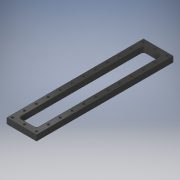
# Autodesk Inventor part: PVCmiddle
Saved by Autodesk Inventor 2019.4 (Build 234330000, 330)
## iProperties
Created: 2020-04-27
Part Number: PVCmiddle
Material: Generic
Document SubType Name: Modeling
Designer: Ed
Density: 1 g/cm^3
Appearance: Default
Author: Ed
Autodesk Inventor part; units mm, degrees
ref_plane "YZ Plane" through (0, 0, 0) normal (1, 0, 0) x (0, 1, 0)
ref_plane "XZ Plane" through (0, 0, 0) normal (0, 1, 0) x (-1, 0, 0)
ref_plane "XY Plane" through (0, 0, 0) normal (0, 0, 1) x (1, 0, 0)
sketch "Sketch1" plane through (0, 0, 0) normal (0, 1, 0) x (-1, 0, 0)
  line L0 (135.3948, 0) -> (136.2838, 0)
  arc A0 (162.481, 269.4826) -> (164.973, 271.8943) centre (162.56, 271.8943) ccw
  arc A1 (164.973, 271.8943) -> (164.8183, 272.7443) centre (162.56, 271.8943) ccw
  arc A2 (164.8183, 272.7443) -> (163.1941, 274.2225) centre (162.56, 271.8943) ccw
  arc A3 (163.1941, 274.2225) -> (162.7264, 274.3016) centre (162.56, 271.8943) ccw
  arc A4 (162.7264, 274.3016) -> (160.2292, 272.5188) centre (162.56, 271.8943) ccw
  arc A5 (160.2292, 272.5188) -> (160.147, 271.8943) centre (162.56, 271.8943) ccw
  arc A6 (160.147, 271.8943) -> (161.9355, 269.5635) centre (162.56, 271.8943) ccw
  arc A7 (161.9355, 269.5635) -> (162.481, 269.4826) centre (162.56, 271.8943) ccw
  arc A8 (162.3235, 242.9385) -> (164.2662, 243.6336) centre (162.56, 245.3399) ccw
  arc A9 (164.2662, 243.6336) -> (164.973, 245.3399) centre (162.56, 245.3399) ccw
  arc A10 (164.973, 245.3399) -> (162.7965, 247.7413) centre (162.56, 245.3399) ccw
  arc A11 (162.7965, 247.7413) -> (160.8538, 247.0461) centre (162.56, 245.3399) ccw
  arc A12 (160.8538, 247.0461) -> (160.147, 245.3399) centre (162.56, 245.3399) ccw
  arc A13 (160.147, 245.3399) -> (162.3235, 242.9385) centre (162.56, 245.3399) ccw
  arc A14 (162.481, 216.3737) -> (164.973, 218.7854) centre (162.56, 218.7854) ccw
  arc A15 (164.973, 218.7854) -> (164.8691, 219.4859) centre (162.56, 218.7854) ccw
  arc A16 (164.8691, 219.4859) -> (163.1463, 221.1261) centre (162.56, 218.7854) ccw
  arc A17 (163.1463, 221.1261) -> (162.5304, 221.1983) centre (162.56, 218.7854) ccw
  arc A18 (162.5304, 221.1983) -> (160.8538, 220.4917) centre (162.56, 218.7854) ccw
  arc A19 (160.8538, 220.4917) -> (160.147, 218.7854) centre (162.56, 218.7854) ccw
  arc A20 (160.147, 218.7854) -> (161.9355, 216.4547) centre (162.56, 218.7854) ccw
  arc A21 (161.9355, 216.4547) -> (162.481, 216.3737) centre (162.56, 218.7854) ccw
  arc A22 (162.3235, 189.8296) -> (164.2662, 190.5248) centre (162.56, 192.231) ccw
  arc A23 (164.2662, 190.5248) -> (164.973, 192.231) centre (162.56, 192.231) ccw
  arc A24 (164.973, 192.231) -> (163.1845, 194.5618) centre (162.56, 192.231) ccw
  arc A25 (163.1845, 194.5618) -> (162.7178, 194.6388) centre (162.56, 192.231) ccw
  arc A26 (162.7178, 194.6388) -> (161.3535, 194.3207) centre (162.56, 192.231) ccw
  arc A27 (161.3535, 194.3207) -> (160.147, 192.231) centre (162.56, 192.231) ccw
  arc A28 (160.147, 192.231) -> (162.3235, 189.8296) centre (162.56, 192.231) ccw
  arc A29 (162.481, 163.2649) -> (164.973, 165.6766) centre (162.56, 165.6766) ccw
  arc A30 (164.973, 165.6766) -> (164.6497, 166.8831) centre (162.56, 165.6766) ccw
  arc A31 (164.6497, 166.8831) -> (162.7178, 168.0844) centre (162.56, 165.6766) ccw
  arc A32 (162.7178, 168.0844) -> (161.3535, 167.7663) centre (162.56, 165.6766) ccw
  arc A33 (161.3535, 167.7663) -> (160.147, 165.6766) centre (162.56, 165.6766) ccw
  arc A34 (160.147, 165.6766) -> (161.9355, 163.3458) centre (162.56, 165.6766) ccw
  arc A35 (161.9355, 163.3458) -> (162.481, 163.2649) centre (162.56, 165.6766) ccw
  arc A36 (162.3235, 136.7208) -> (164.2662, 137.4159) centre (162.56, 139.1221) ccw
  arc A37 (164.2662, 137.4159) -> (164.973, 139.1222) centre (162.56, 139.1221) ccw
  arc A38 (164.973, 139.1222) -> (163.1845, 141.4529) centre (162.56, 139.1221) ccw
  arc A39 (163.1845, 141.4529) -> (162.7178, 141.53) centre (162.56, 139.1221) ccw
  arc A40 (162.7178, 141.53) -> (161.3535, 141.2119) centre (162.56, 139.1221) ccw
  arc A41 (161.3535, 141.2119) -> (160.147, 139.1222) centre (162.56, 139.1221) ccw
  arc A42 (160.147, 139.1222) -> (162.3235, 136.7208) centre (162.56, 139.1221) ccw
  arc A43 (162.481, 110.156) -> (164.973, 112.5677) centre (162.56, 112.5677) ccw
  arc A44 (164.973, 112.5677) -> (164.7242, 113.635) centre (162.56, 112.5677) ccw
  arc A45 (164.7242, 113.635) -> (162.7572, 114.9726) centre (162.56, 112.5677) ccw
  arc A46 (162.7572, 114.9726) -> (161.9355, 114.8985) centre (162.56, 112.5677) ccw
  arc A47 (161.9355, 114.8985) -> (160.147, 112.5677) centre (162.56, 112.5677) ccw
  arc A48 (160.147, 112.5677) -> (161.9355, 110.2369) centre (162.56, 112.5677) ccw
  arc A49 (161.9355, 110.2369) -> (162.481, 110.156) centre (162.56, 112.5677) ccw
  arc A50 (162.7178, 83.6055) -> (164.6497, 84.8068) centre (162.56, 86.0133) ccw
  arc A51 (164.6497, 84.8068) -> (164.973, 86.0133) centre (162.56, 86.0133) ccw
  arc A52 (164.973, 86.0133) -> (163.0308, 88.3799) centre (162.56, 86.0133) ccw
  arc A53 (163.0308, 88.3799) -> (162.7572, 88.4182) centre (162.56, 86.0133) ccw
  arc A54 (162.7572, 88.4182) -> (161.9355, 88.3441) centre (162.56, 86.0133) ccw
  arc A55 (161.9355, 88.3441) -> (160.147, 86.0133) centre (162.56, 86.0133) ccw
  arc A56 (160.147, 86.0133) -> (161.9355, 83.6825) centre (162.56, 86.0133) ccw
  arc A57 (161.9355, 83.6825) -> (162.7178, 83.6055) centre (162.56, 86.0133) ccw
  arc A58 (162.481, 57.0472) -> (164.973, 59.4589) centre (162.56, 59.4589) ccw
  arc A59 (164.973, 59.4589) -> (164.4253, 60.9897) centre (162.56, 59.4589) ccw
  arc A60 (164.4253, 60.9897) -> (162.6192, 61.8711) centre (162.56, 59.4589) ccw
  arc A61 (162.6192, 61.8711) -> (161.9355, 61.7896) centre (162.56, 59.4589) ccw
  arc A62 (161.9355, 61.7896) -> (160.147, 59.4589) centre (162.56, 59.4589) ccw
  arc A63 (160.147, 59.4589) -> (161.9355, 57.1281) centre (162.56, 59.4589) ccw
  arc A64 (161.9355, 57.1281) -> (162.481, 57.0472) centre (162.56, 59.4589) ccw
  arc A65 (162.7178, 30.4966) -> (164.6497, 31.6979) centre (162.56, 32.9044) ccw
  arc A66 (164.6497, 31.6979) -> (164.973, 32.9044) centre (162.56, 32.9044) ccw
  arc A67 (164.973, 32.9044) -> (163.0308, 35.2711) centre (162.56, 32.9044) ccw
  arc A68 (163.0308, 35.2711) -> (162.7572, 35.3094) centre (162.56, 32.9044) ccw
  arc A69 (162.7572, 35.3094) -> (161.9355, 35.2352) centre (162.56, 32.9044) ccw
  arc A70 (161.9355, 35.2352) -> (160.147, 32.9044) centre (162.56, 32.9044) ccw
  arc A71 (160.147, 32.9044) -> (161.9355, 30.5737) centre (162.56, 32.9044) ccw
  arc A72 (161.9355, 30.5737) -> (162.7178, 30.4966) centre (162.56, 32.9044) ccw
  arc A73 (160.147, 6.35) -> (164.973, 6.35) centre (162.56, 6.35) ccw
  arc A74 (164.973, 6.35) -> (164.4253, 7.8808) centre (162.56, 6.35) ccw
  arc A75 (164.4253, 7.8808) -> (162.6192, 8.7623) centre (162.56, 6.35) ccw
  arc A76 (162.6192, 8.7623) -> (161.9355, 8.6808) centre (162.56, 6.35) ccw
  arc A77 (161.9355, 8.6808) -> (160.147, 6.35) centre (162.56, 6.35) ccw
  arc A78 (133.477, 6.35) -> (138.2208, 5.7255) centre (135.89, 6.35) ccw
  arc A79 (138.2208, 5.7255) -> (138.2824, 6.035) centre (135.89, 6.35) ccw
  arc A80 (138.2824, 6.035) -> (138.2978, 6.1922) centre (135.89, 6.35) ccw
  arc A81 (138.2978, 6.1922) -> (138.303, 6.35) centre (135.89, 6.35) ccw
  arc A82 (138.303, 6.35) -> (135.2655, 8.6808) centre (135.89, 6.35) ccw
  arc A83 (135.2655, 8.6808) -> (133.477, 6.35) centre (135.89, 6.35) ccw
  arc A84 (109.22, 8.763) -> (107.8794, 8.3563) centre (109.22, 6.35) ccw
  arc A85 (107.8794, 8.3563) -> (106.807, 6.35) centre (109.22, 6.35) ccw
  arc A86 (106.807, 6.35) -> (111.1814, 4.9445) centre (109.22, 6.35) ccw
  arc A87 (111.1814, 4.9445) -> (111.5508, 5.7255) centre (109.22, 6.35) ccw
  arc A88 (111.5508, 5.7255) -> (111.6278, 6.1922) centre (109.22, 6.35) ccw
  arc A89 (111.6278, 6.1922) -> (111.633, 6.35) centre (109.22, 6.35) ccw
  arc A90 (111.633, 6.35) -> (109.22, 8.763) centre (109.22, 6.35) ccw
  arc A91 (109.3088, 35.3158) -> (109.22, 35.3174) centre (109.22, 32.9044) ccw
  arc A92 (109.22, 35.3174) -> (106.807, 32.9044) centre (109.22, 32.9044) ccw
  arc A93 (106.807, 32.9044) -> (108.5955, 30.5737) centre (109.22, 32.9044) ccw
  arc A94 (108.5955, 30.5737) -> (109.141, 30.4927) centre (109.22, 32.9044) ccw
  arc A95 (109.141, 30.4927) -> (111.633, 32.9044) centre (109.22, 32.9044) ccw
  arc A96 (111.633, 32.9044) -> (109.6908, 35.2711) centre (109.22, 32.9044) ccw
  arc A97 (109.6908, 35.2711) -> (109.5741, 35.2913) centre (109.22, 32.9044) ccw
  arc A98 (109.5741, 35.2913) -> (109.3088, 35.3158) centre (109.22, 32.9044) ccw
  arc A99 (109.3384, 61.869) -> (109.22, 61.8719) centre (109.22, 59.4589) ccw
  arc A100 (109.22, 61.8719) -> (107.8794, 61.4652) centre (109.22, 59.4589) ccw
  arc A101 (107.8794, 61.4652) -> (106.807, 59.4589) centre (109.22, 59.4589) ccw
  arc A102 (106.807, 59.4589) -> (108.5955, 57.1281) centre (109.22, 59.4589) ccw
  arc A103 (108.5955, 57.1281) -> (109.141, 57.0472) centre (109.22, 59.4589) ccw
  arc A104 (109.141, 57.0472) -> (111.633, 59.4589) centre (109.22, 59.4589) ccw
  arc A105 (111.633, 59.4589) -> (109.6908, 61.8255) centre (109.22, 59.4589) ccw
  arc A106 (109.6908, 61.8255) -> (109.3384, 61.869) centre (109.22, 59.4589) ccw
  arc A107 (109.3088, 88.4247) -> (109.22, 88.4263) centre (109.22, 86.0133) ccw
  arc A108 (109.22, 88.4263) -> (106.807, 86.0133) centre (109.22, 86.0133) ccw
  arc A109 (106.807, 86.0133) -> (108.5955, 83.6825) centre (109.22, 86.0133) ccw
  arc A110 (108.5955, 83.6825) -> (109.141, 83.6016) centre (109.22, 86.0133) ccw
  arc A111 (109.141, 83.6016) -> (111.633, 86.0133) centre (109.22, 86.0133) ccw
  arc A112 (111.633, 86.0133) -> (109.6908, 88.3799) centre (109.22, 86.0133) ccw
  arc A113 (109.6908, 88.3799) -> (109.5741, 88.4002) centre (109.22, 86.0133) ccw
  arc A114 (109.5741, 88.4002) -> (109.3088, 88.4247) centre (109.22, 86.0133) ccw
  arc A115 (109.3384, 114.9778) -> (109.22, 114.9807) centre (109.22, 112.5677) ccw
  arc A116 (109.22, 114.9807) -> (107.5138, 114.274) centre (109.22, 112.5677) ccw
  arc A117 (107.5138, 114.274) -> (106.807, 112.5677) centre (109.22, 112.5677) ccw
  arc A118 (106.807, 112.5677) -> (108.5955, 110.2369) centre (109.22, 112.5677) ccw
  arc A119 (108.5955, 110.2369) -> (109.141, 110.156) centre (109.22, 112.5677) ccw
  arc A120 (109.141, 110.156) -> (111.633, 112.5677) centre (109.22, 112.5677) ccw
  arc A121 (111.633, 112.5677) -> (109.6908, 114.9344) centre (109.22, 112.5677) ccw
  arc A122 (109.6908, 114.9344) -> (109.3384, 114.9778) centre (109.22, 112.5677) ccw
  arc A123 (109.3088, 141.5335) -> (109.22, 141.5352) centre (109.22, 139.1222) ccw
  arc A124 (109.22, 141.5352) -> (106.807, 139.1222) centre (109.22, 139.1222) ccw
  arc A125 (106.807, 139.1222) -> (108.5955, 136.7914) centre (109.22, 139.1222) ccw
  arc A126 (108.5955, 136.7914) -> (109.141, 136.7104) centre (109.22, 139.1222) ccw
  arc A127 (109.141, 136.7104) -> (111.633, 139.1222) centre (109.22, 139.1222) ccw
  arc A128 (111.633, 139.1222) -> (109.6908, 141.4888) centre (109.22, 139.1222) ccw
  arc A129 (109.6908, 141.4888) -> (109.5741, 141.509) centre (109.22, 139.1222) ccw
  arc A130 (109.5741, 141.509) -> (109.3088, 141.5335) centre (109.22, 139.1222) ccw
  arc A131 (109.3384, 168.0867) -> (109.22, 168.0896) centre (109.22, 165.6766) ccw
  arc A132 (109.22, 168.0896) -> (107.5138, 167.3828) centre (109.22, 165.6766) ccw
  arc A133 (107.5138, 167.3828) -> (106.807, 165.6766) centre (109.22, 165.6766) ccw
  arc A134 (106.807, 165.6766) -> (108.5955, 163.3458) centre (109.22, 165.6766) ccw
  arc A135 (108.5955, 163.3458) -> (109.141, 163.2649) centre (109.22, 165.6766) ccw
  arc A136 (109.141, 163.2649) -> (111.633, 165.6766) centre (109.22, 165.6766) ccw
  arc A137 (111.633, 165.6766) -> (109.6908, 168.0432) centre (109.22, 165.6766) ccw
  arc A138 (109.6908, 168.0432) -> (109.3384, 168.0867) centre (109.22, 165.6766) ccw
  arc A139 (109.4172, 194.6359) -> (108.5955, 194.5618) centre (109.22, 192.231) ccw
  arc A140 (108.5955, 194.5618) -> (106.807, 192.231) centre (109.22, 192.231) ccw
  arc A141 (106.807, 192.231) -> (108.5955, 189.9002) centre (109.22, 192.231) ccw
  arc A142 (108.5955, 189.9002) -> (109.141, 189.8193) centre (109.22, 192.231) ccw
  arc A143 (109.141, 189.8193) -> (111.633, 192.231) centre (109.22, 192.231) ccw
  arc A144 (111.633, 192.231) -> (109.6908, 194.5976) centre (109.22, 192.231) ccw
  arc A145 (109.6908, 194.5976) -> (109.4172, 194.6359) centre (109.22, 192.231) ccw
  arc A146 (109.4172, 221.1904) -> (108.5955, 221.1162) centre (109.22, 218.7854) ccw
  arc A147 (108.5955, 221.1162) -> (107.3056, 220.2544) centre (109.22, 218.7854) ccw
  arc A148 (107.3056, 220.2544) -> (106.807, 218.7854) centre (109.22, 218.7854) ccw
  arc A149 (106.807, 218.7854) -> (108.5955, 216.4547) centre (109.22, 218.7854) ccw
  arc A150 (108.5955, 216.4547) -> (109.141, 216.3737) centre (109.22, 218.7854) ccw
  arc A151 (109.141, 216.3737) -> (111.633, 218.7854) centre (109.22, 218.7854) ccw
  arc A152 (111.633, 218.7854) -> (109.6908, 221.1521) centre (109.22, 218.7854) ccw
  arc A153 (109.6908, 221.1521) -> (109.4172, 221.1904) centre (109.22, 218.7854) ccw
  arc A154 (109.6228, 242.9607) -> (111.633, 245.3399) centre (109.22, 245.3399) ccw
  arc A155 (111.633, 245.3399) -> (110.4605, 247.4096) centre (109.22, 245.3399) ccw
  arc A156 (110.4605, 247.4096) -> (109.6908, 247.7065) centre (109.22, 245.3399) ccw
  arc A157 (109.6908, 247.7065) -> (108.5955, 247.6706) centre (109.22, 245.3399) ccw
  arc A158 (108.5955, 247.6706) -> (106.807, 245.3399) centre (109.22, 245.3399) ccw
  arc A159 (106.807, 245.3399) -> (108.5955, 243.0091) centre (109.22, 245.3399) ccw
  arc A160 (108.5955, 243.0091) -> (109.141, 242.9282) centre (109.22, 245.3399) ccw
  arc A161 (109.141, 242.9282) -> (109.6228, 242.9607) centre (109.22, 245.3399) ccw
  line L1 (115.57, 263.784) -> (115.57, 255.017)
  line L2 (115.57, 255.017) -> (115.57, 252.4125)
  line L3 (115.57, 252.4125) -> (115.57, 19.05)
  arc A162 (115.57, 19.05) -> (121.92, 12.7) centre (121.92, 19.05) ccw
  line L4 (121.92, 12.7) -> (149.86, 12.7)
  arc A163 (149.86, 12.7) -> (156.21, 19.05) centre (149.86, 19.05) ccw
  line L5 (156.21, 19.05) -> (156.21, 47.8145)
  line L6 (156.21, 49.3385) -> (156.21, 285.75)
  arc A164 (156.21, 285.75) -> (149.86, 292.1) centre (149.86, 285.75) ccw
  line L7 (149.86, 292.1) -> (121.92, 292.1)
  arc A165 (121.92, 292.1) -> (115.57, 285.75) centre (121.92, 285.75) ccw
  line L8 (115.57, 285.75) -> (115.57, 273.2484)
  line L9 (115.57, 273.2484) -> (115.57, 265.308)
  arc A166 (109.3778, 274.3021) -> (108.0135, 273.984) centre (109.22, 271.8943) ccw
  arc A167 (108.0135, 273.984) -> (107.1303, 273.1008) centre (109.22, 271.8943) ccw
  arc A168 (107.1303, 273.1008) -> (106.807, 271.8943) centre (109.22, 271.8943) ccw
  arc A169 (106.807, 271.8943) -> (108.7492, 269.5277) centre (109.22, 271.8943) ccw
  arc A170 (108.7492, 269.5277) -> (109.22, 269.4813) centre (109.22, 271.8943) ccw
  arc A171 (109.22, 269.4813) -> (110.5606, 269.888) centre (109.22, 271.8943) ccw
  arc A172 (110.5606, 269.888) -> (111.633, 271.8943) centre (109.22, 271.8943) ccw
  arc A173 (111.633, 271.8943) -> (109.8445, 274.2251) centre (109.22, 271.8943) ccw
  arc A174 (109.8445, 274.2251) -> (109.3778, 274.3021) centre (109.22, 271.8943) ccw
  arc A175 (111.633, 298.4487) -> (107.2586, 299.8542) centre (109.22, 298.4487) ccw
  arc A176 (107.2586, 299.8542) -> (106.8892, 299.0733) centre (109.22, 298.4487) ccw
  arc A177 (106.8892, 299.0733) -> (106.807, 298.4487) centre (109.22, 298.4487) ccw
  arc A178 (106.807, 298.4487) -> (107.5138, 296.7425) centre (109.22, 298.4487) ccw
  arc A179 (107.5138, 296.7425) -> (108.7492, 296.0821) centre (109.22, 298.4487) ccw
  arc A180 (108.7492, 296.0821) -> (111.633, 298.4487) centre (109.22, 298.4487) ccw
  arc A181 (138.2978, 298.2922) -> (138.303, 298.45) centre (135.89, 298.45) ccw
  arc A182 (138.303, 298.45) -> (133.5592, 299.0745) centre (135.89, 298.45) ccw
  arc A183 (133.5592, 299.0745) -> (133.4976, 298.765) centre (135.89, 298.45) ccw
  arc A184 (133.4976, 298.765) -> (133.4822, 298.6078) centre (135.89, 298.45) ccw
  arc A185 (133.4822, 298.6078) -> (133.477, 298.45) centre (135.89, 298.45) ccw
  arc A186 (133.477, 298.45) -> (138.2208, 297.8255) centre (135.89, 298.45) ccw
  arc A187 (138.2208, 297.8255) -> (138.2824, 298.135) centre (135.89, 298.45) ccw
  arc A188 (138.2824, 298.135) -> (138.2978, 298.2922) centre (135.89, 298.45) ccw
  arc A189 (164.973, 298.4487) -> (160.2292, 299.0733) centre (162.56, 298.4487) ccw
  arc A190 (160.2292, 299.0733) -> (160.1676, 298.7637) centre (162.56, 298.4487) ccw
  arc A191 (160.1676, 298.7637) -> (160.147, 298.4487) centre (162.56, 298.4487) ccw
  arc A192 (160.147, 298.4487) -> (161.9355, 296.118) centre (162.56, 298.4487) ccw
  arc A193 (161.9355, 296.118) -> (163.7665, 296.359) centre (162.56, 298.4487) ccw
  arc A194 (163.7665, 296.359) -> (164.973, 298.4487) centre (162.56, 298.4487) ccw
  line L10 (102.87, 0) -> (135.3948, 0)
  line L11 (102.87, 304.8) -> (102.87, 0)
  line L12 (168.91, 304.8) -> (102.87, 304.8)
  line L13 (168.91, 0) -> (168.91, 304.8)
  line L14 (136.2838, 0) -> (168.91, 0)
  line L15 (115.57, 265.308) -> (115.57, 263.784)
  line L16 (156.21, 49.3385) -> (156.21, 47.8145)
  constraints: 390 point on circle, 195 centre point, 34 end point, 13 tangent, 3 collinear, 1 parallel
extrude "Extrusion1" add sketch "Sketch1" along normal blind 12.7
body "Solid1"
